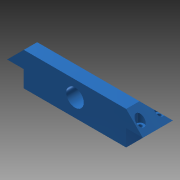
# Autodesk Inventor part: ZAxisNutMount
Saved by Autodesk Inventor 2015 SP1 (Build 190203100, 203)
## iProperties
Created: 2014-12-11
Part Number: ZAxisNutMount
Material: Generic
Document SubType Name: Modeling
Designer: Jack
Density: 1 g/cm^3
Appearance: Cyan
Mass: 40.457 g
Surface Area: 119.041 cm^2
Volume: 40.457 cm^3
Author: Jack
Autodesk Inventor part; units mm, degrees
ref_plane "YZ Plane" through (0, 0, 0) normal (1, 0, 0) x (0, 1, 0)
sketch "Sketch1" plane through (0, 0, 0) normal (0, 0, 1) x (1, 0, 0)
  line L0 (0, 0) -> (92, 0)
  line L1 (92, 0) -> (92, 12)
  line L2 (92, 12) -> (0, 12)
  line L3 (0, 12) -> (0, 0)
  dimension "d0" = 92
  dimension "d1" = 12
  constraints: 8 end point, 2 parallel, 1 horizontal, 1 perpendicular
  measures "d0" distance of L2.end L1.end
  measures "d1" distance of L2.end L0.start
extrude "Extrusion1" add sketch "Sketch1" along normal blind 30
sketch "Sketch3" plane through (0, 12, 30) normal (0, 1, 0) x (1, 0, 0)
  line L0 (0, 30) -> (0, 0) projected
  line L1 (92, 30) -> (0, 30) projected
  circle A0 centre (46, 14.15) radius 7.9
  point P0 (0, 17)
  point P1 (107, 32)
  point P2 (15, 32)
  dimension "d8" = 15.8
  dimension "d9" = 15.85
  dimension "d10" = 46
  constraints: 1 centre point, 1 other
  measures "d8" diameter of A0
  measures "d10" distance from line of L0 A0.centre
extrude "Extrusion3" cut sketch "Sketch3" against normal up to next
sketch "Sketch4" plane through (0, 12, 0) normal (0, 1, 0) x (1, 0, 0)
  line L0 (0, 0) -> (0, -30) projected
  line L1 (92, 0) -> (92, -30) projected
  line L2 (0, -30) -> (-15, -15)
  line L3 (-15, -15) -> (0, -15)
  line L4 (92, -30) -> (107, -15)
  line L5 (107, -15) -> (92, -15)
  dimension "d13" = 45
  dimension "d14" = 45
  constraints: 8 end point, 2 midpoint, 1 perpendicular, 1 point on line
  measures "d13" angle of L1 L4
  measures "d14" angle of L0 L2
extrude "Extrusion4" add sketch "Sketch4" against normal up to surface (12 mm away)
sketch "Sketch5" plane through (0, 0, 0) normal (1, 0, 0) x (0, 1, 0)
  line L0 (0, 15) -> (0, 30) projected
  line L1 (12, 30) -> (0, 30) projected
  line L2 (12, 15) -> (12, 30) projected
  line L3 (12, 15) -> (0, 15) projected
  line L4 (12, 15) -> (27, 15)
  line L5 (27, 15) -> (12, 30)
  point P0 (0, 0)
  dimension "d17" = 15
  constraints: 4 end point, 1 horizontal
  measures "d17" distance of L2.start L4.end
extrude "Extrusion5" add sketch "Sketch5" against normal up to surface contours L2 L5 L4 surface through (0, 12, 30) normal (-0.7071, 0, 0.7071)
sketch "Sketch6" plane through (92, 0, 0) normal (1, 0, 0) x (0, 0, -1)
  line L0 (-30, 0) -> (-15, 0) projected
  line L1 (-15, 12) -> (-15, 0) projected
  line L2 (-30, 12) -> (-15, 12) projected
  line L3 (-30, 0) -> (-30, 12) projected
  line L4 (-15, 12) -> (-15, 27)
  line L5 (-15, 27) -> (-30, 12)
  dimension "d20" = 15
  constraints: 4 end point, 1 vertical
  measures "d20" distance of L1.start L4.end
extrude "Extrusion6" add sketch "Sketch6" along normal up to surface contours L5 L4 L2 surface through (107, 12, 15) normal (0.7071, 0, 0.7071)
sketch "Sketch7" plane through (0, 0, 0) normal (0, 0, -1) x (-1, 0, 0)
  line L0 (-92, 12) -> (0, 12) projected
  line L1 (-92, 12) -> (-92, 27)
  line L2 (-92, 27) -> (-77, 12)
  line L3 (0, 12) -> (0, 27)
  line L4 (0, 27) -> (-15, 12)
  dimension "d23" = 15
  dimension "d24" = 15
  constraints: 8 end point, 2 point on line, 2 vertical, 1 horizontal alignment, 1 perpendicular
  measures "d23" distance of L0.start L1.end
  measures "d24" distance of L0.start L2.end
extrude "Extrusion7" add sketch "Sketch7" against normal up to surface surface through (92, 27, 15) normal (0, 0.7071, 0.7071)
sketch "Sketch8" plane through (0, 0, 30) normal (0, 0, 1) x (1, 0, 0)
  line L0 (-15, 0) -> (0, 0) projected
  line L1 (0, 12) -> (0, 0) projected
  line L2 (-15, 27) -> (0, 12) projected
  line L3 (-15, 0) -> (-15, 27) projected
  line L4 (92, 0) -> (107, 0) projected
  line L5 (107, 27) -> (107, 0) projected
  line L6 (92, 12) -> (107, 27) projected
  line L7 (92, 0) -> (92, 12) projected
  circle A0 centre (-7.5, 5) radius 1.75
  circle A1 centre (-7.5, 22) radius 1.75
  circle A2 centre (99.5, 22) radius 1.75
  circle A3 centre (99.5, 5) radius 1.75
  line L8 (92, 27) -> (107, 27) projected
  dimension "d27" = 3.5
  dimension "d28" = 7.5
  dimension "d29" = 7.5
  dimension "d30" = 5
  dimension "d31" = 5
  constraints: 4 centre point, 3 equal radius, 2 horizontal alignment, 2 vertical alignment
  measures "d27" diameter of A0
  measures "d28" distance from line of L3 A0.centre
  measures "d29" distance from line of L5 A3.centre
  measures "d30" distance from line of L4 A3.centre
  measures "d31" distance from line of L8 A2.centre
extrude "Extrusion8" cut sketch "Sketch8" against normal up to surface (15 mm away) contours A0 | A1 | A2 | A3
sketch "Sketch9" plane through (0, 0, 30) normal (0, 0, 1) x (1, 0, 0)
  circle A0 centre (-7.5, 22) radius 1.75 projected
  circle A1 centre (-7.5, 5) radius 1.75 projected
  circle A2 centre (99.5, 22) radius 1.75 projected
  circle A3 centre (99.5, 5) radius 1.75 projected
  circle A4 centre (-7.5, 22) radius 3.65
  circle A5 centre (-7.5, 5) radius 3.65
  circle A6 centre (99.5, 22) radius 3.65
  circle A7 centre (99.5, 5) radius 3.65
  dimension "d34" = 7.3
  constraints: 4 centre point, 4 coincident, 3 equal radius
  measures "d34" diameter of A4
extrude "Extrusion9" cut sketch "Sketch9" against normal blind 12
ref_plane "Work Plane1" through (77, 0, 15) normal (1, 0, 0) x (0, 0, -1)
sketch "Sketch10" plane through (77, 0, 15) normal (1, 0, 0) x (0, 0, -1)
  line L0 (-15, 12) -> (0, 27) projected
  line L1 (15, 27) -> (0, 27) projected
  line L2 (15, 12) -> (15, 27) projected
  line L3 (-15, 12) -> (15, 12) projected
  circle A0 centre (7.5, 22) radius 1.75
  circle A1 centre (7.5, 22) radius 3.65
  point P0 (15, 0)
  dimension "d38" = 3.5
  dimension "d39" = 7.3
  dimension "d40" = 5
  dimension "d41" = 7.5
  constraints: 2 centre point, 1 coincident
  measures "d38" diameter of A0
  measures "d39" diameter of A1
  measures "d40" distance from line of L1 A0.centre
  measures "d41" distance from line of L2 A0.centre
extrude "Extrusion10" cut sketch "Sketch10" along normal up to surface (15 mm away) contours A0
sketch "Sketch11" plane through (77, 0, 15) normal (1, 0, 0) x (0, 0, -1)
  circle A0 centre (7.5, 22) radius 1.75 projected
  circle A1 centre (7.5, 22) radius 3.65
  point P0 (15, 0)
  dimension "d44" = 7.3
  constraints: 1 centre point, 1 coincident
  measures "d44" diameter of A1
extrude "Extrusion11" cut sketch "Sketch11" along normal blind 12
ref_plane "Work Plane2" through (15, 0, 0) normal (-1, 0, 0) x (0, 0, 1)
sketch "Sketch12" plane through (15, 0, 0) normal (-1, 0, 0) x (0, 0, 1)
  line L0 (15, 27) -> (30, 12) projected
  line L1 (0, 12) -> (30, 12) projected
  line L2 (0, 27) -> (0, 12) projected
  line L3 (0, 27) -> (15, 27) projected
  circle A0 centre (7.5, 22) radius 1.75
  point P0 (0, 0)
  dimension "d48" = 3.5
  dimension "d49" = 7.5
  dimension "d50" = 5
  constraints: 1 centre point
  measures "d48" diameter of A0
  measures "d49" distance from line of L2 A0.centre
  measures "d50" distance from line of L3 A0.centre
extrude "Extrusion12" cut sketch "Sketch12" along normal up to surface (15 mm away) contours A0
sketch "Sketch13" plane through (15, 0, 0) normal (-1, 0, 0) x (0, 0, 1)
  circle A0 centre (7.5, 22) radius 1.75 projected
  circle A1 centre (7.5, 22) radius 1.75 projected
  circle A2 centre (7.5, 22) radius 3.65
  point P0 (0, 0)
  dimension "d53" = 7.3
  constraints: 1 centre point, 1 coincident
  measures "d53" diameter of A2
extrude "Extrusion13" cut sketch "Sketch13" along normal blind 12
body "Solid1"
